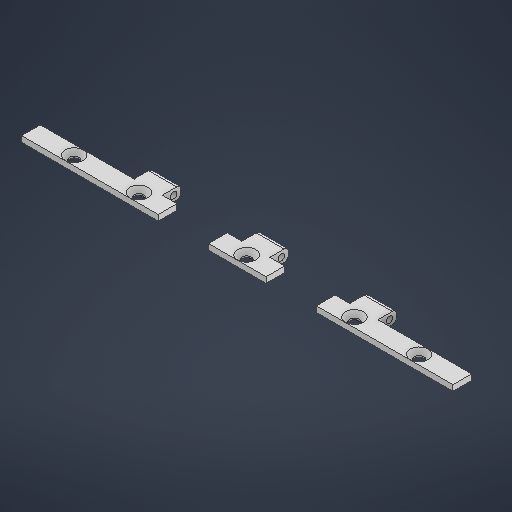
# Autodesk Inventor part: mocowanie do pługu
Saved by Autodesk Inventor 2026.2 (Build 302298010, 298A)
## iProperties
Created: 2026-05-09
Part Number: mocowanie do pługu
Material: Ogólny
Document SubType Name: Modeling
Designer: karol
Density: 1 g/cm^3
Appearance: Domyślna
Author: karol
Autodesk Inventor part; units mm, degrees
ref_plane "YZ Plane" through (0, 0, 0) normal (1, 0, 0) x (0, 1, 0)
ref_plane "XZ Plane" through (0, 0, 0) normal (0, 1, 0) x (-1, 0, 0)
ref_plane "XY Plane" through (0, 0, 0) normal (0, 0, 1) x (1, 0, 0)
sketch "Szkic1" plane through (0, 0, 0) normal (0, 1, 0) x (-1, 0, 0)
  line L0 (0, 0) -> (-4.9, 0)
  line L1 (-4.9, 0) -> (4.9, 0)
  line L2 (4.9, 0) -> (-4.8, 0)
  line L3 (-4.8, 0) -> (-4.8, -4.8)
  line L4 (-4.8, -4.8) -> (4.9, -4.8)
  line L5 (4.9, -4.8) -> (4.9, 0)
  line L6 (0, 0) -> (-37.5, 0)
  line L7 (0, 0) -> (37.5, 0)
  line L8 (37.5, 0) -> (32.6, 0)
  line L9 (37.5, 0) -> (42.4, 0)
  line L10 (-37.5, 0) -> (-32.6, 0)
  line L11 (-32.6, 0) -> (-42.4, 0)
  line L12 (42.4, 0) -> (32.6, 0)
  line L13 (32.6, 0) -> (32.6, -4.8)
  line L14 (32.6, -4.8) -> (42.4, -4.8)
  line L15 (42.4, -4.8) -> (42.4, 0)
  line L16 (-32.6, 0) -> (-42.4, 0)
  line L17 (-42.4, 0) -> (-42.4, -4.8)
  line L18 (-42.4, -4.8) -> (-32.6, -4.8)
  line L19 (-32.6, -4.8) -> (-32.6, 0)
  point P0 (-4.8, 0)
  dimension "d0" = 4.9
  dimension "d1" = 9.8
  dimension "d2" = 4.8
  dimension "d3" = 37.5
  dimension "d4" = 37.5
  dimension "d5" = 4.9
  dimension "d6" = 4.9
  dimension "d7" = 4.9
  dimension "d8" = 9.8
  constraints: 40 end point, 7 point on line, 6 parallel, 5 horizontal, 3 perpendicular
  measures "d0" distance of L0.start L0.end
  measures "d1" distance of L0.end L1.end
  measures "d2" distance of L3.end L2.end
  measures "d3" distance of L0.start L6.end
  measures "d4" distance of L0.start L7.end
  measures "d5" distance of L7.end L8.end
  measures "d6" distance of L7.end L9.end
  measures "d7" distance of L6.end L10.end
  measures "d8" distance of L10.end L11.end
extrude "Wyciągnięcie proste1" add sketch "Szkic1" along normal blind 4
sketch "Szkic2" plane through (-32.6, 0, 0) normal (1, 0, 0) x (0, 0, -1)
  circle A0 centre (2.4, 2) radius 1.15
  line L0 (0, 4) -> (4.8, 4) projected
  line L1 (4.8, 0) -> (4.8, 4) projected
  point P0 (0, 0)
  dimension "d11" = 2.3
  dimension "d12" = 2
  dimension "d13" = 2.4
  constraints: 1 centre point
  measures "d11" diameter of A0
  measures "d12" distance from line of L0 A0.centre
  measures "d13" distance from line of L1 A0.centre
sketch "Szkic3" plane through (4.8, 0, 0) normal (1, 0, 0) x (0, 0, -1)
  circle A0 centre (2.4, 2) radius 1.15
  line L0 (4.8, 0) -> (4.8, 4) projected
  line L1 (0, 4) -> (4.8, 4) projected
  point P0 (0, 0)
  dimension "d14" = 2.3
  dimension "d15" = 2.4
  dimension "d16" = 2
  constraints: 1 centre point
  measures "d14" diameter of A0
  measures "d15" distance from line of L0 A0.centre
  measures "d16" distance from line of L1 A0.centre
sketch "Szkic4" plane through (42.4, 0, 0) normal (1, 0, 0) x (0, 0, -1)
  circle A0 centre (2.4, 2) radius 1.15
  line L0 (0, 4) -> (4.8, 4) projected
  line L1 (4.8, 0) -> (4.8, 4) projected
  point P0 (0, 0)
  dimension "d17" = 2.3
  dimension "d18" = 2
  dimension "d19" = 2.4
  constraints: 1 centre point
  measures "d17" diameter of A0
  measures "d18" distance from line of L0 A0.centre
  measures "d19" distance from line of L1 A0.centre
extrude "Wyciągnięcie proste2" cut sketch "Szkic4" against normal blind 9.8
extrude "Wyciągnięcie proste3" cut sketch "Szkic3" against normal blind 9.8
extrude "Wyciągnięcie proste4" cut sketch "Szkic2" against normal blind 9.8
fillet "Zaokrąglenie1" radius 1.25 6 edges at (-0.05, 4, -4.8) (-37.5, 4, -4.8) (37.5, 4, -4.8) (-0.05, 0, -4.8) (37.5, 0, -4.8) (-37.5, 0, -4.8)
sketch "Szkic11" plane through (-42.4, 4, 0) normal (0, 0, 1) x (1, 0, 0)
  line L0 (0, 0) -> (9.8, 0) projected
  line L1 (0, 0) -> (9.8, 0)
  line L2 (9.8, 0) -> (9.8, -4)
  line L3 (9.8, -4) -> (0, -4)
  line L4 (0, -4) -> (0, 0)
  line L5 (37.5, 0) -> (47.2, 0) projected
  line L6 (47.2, -4) -> (47.2, 0) projected
  line L7 (37.5, 0) -> (47.2, 0)
  line L8 (47.2, 0) -> (47.2, -4)
  line L9 (47.2, -4) -> (37.5, -4)
  line L10 (37.5, -4) -> (37.5, 0)
  line L11 (75, 0) -> (84.8, 0) projected
  line L12 (84.8, -4) -> (84.8, 0) projected
  line L13 (75, 0) -> (84.8, 0)
  line L14 (84.8, 0) -> (84.8, -4)
  line L15 (84.8, -4) -> (75, -4)
  line L16 (75, -4) -> (75, 0)
  point P0 (42.4, -4)
  point P1 (47.2, -2)
  point P2 (84.8, -2)
  point P3 (84.8, -2)
  point P4 (47.2, -2)
  constraints: 24 end point, 6 parallel, 3 horizontal, 3 perpendicular
extrude "Wyciągnięcie proste11" add sketch "Szkic11" against normal blind 6.5
sketch "Szkic12" plane through (-42.4, 0, 0) normal (-1, 0, 0) x (0, 0, 1)
  line L0 (0, 4) -> (-6.5, 4) projected
  line L1 (0, 0) -> (-6.5, 0) projected
  line L2 (-6.5, 4) -> (-1.5, 4)
  line L3 (-1.5, 4) -> (-1.5, 0)
  line L4 (-1.5, 0) -> (-6.5, 0)
  line L5 (-6.5, 0) -> (-6.5, 4)
  circle A0 centre (-4, 2) radius 1.1
  point P0 (-6.5, 2)
  dimension "d73" = 5
  dimension "d74" = 2.2
  dimension "d75" = 2
  dimension "d76" = 2.5
  constraints: 8 end point, 2 parallel, 1 centre point, 1 horizontal, 1 midpoint, 1 perpendicular, 1 point on line
  measures "d73" distance of L3.end L4.end
  measures "d74" diameter of A0
  measures "d75" distance from line of L0 A0.centre
  measures "d76" distance of point (-6.5, 2) A0.centre
sketch "Szkic13" plane through (-4.9, 0, 0) normal (-1, 0, 0) x (0, 0, 1)
  line L0 (0, 4) -> (-6.5, 4) projected
  line L1 (0, 0) -> (-6.5, 0) projected
  line L2 (-6.5, 4) -> (-1.5, 4)
  line L3 (-1.5, 4) -> (-1.5, 0)
  line L4 (-1.5, 0) -> (-6.5, 0)
  line L5 (-6.5, 0) -> (-6.5, 4)
  circle A0 centre (-4, 2) radius 1.1
  dimension "d77" = 5
  dimension "d78" = 2.2
  dimension "d79" = 2
  dimension "d80" = 2.5
  constraints: 8 end point, 2 parallel, 1 centre point, 1 horizontal, 1 perpendicular, 1 point on line
  measures "d77" distance of L3.end L4.end
  measures "d78" diameter of A0
  measures "d79" distance from line of L0 A0.centre
  measures "d80" distance from line of L5 A0.centre
sketch "Szkic14" plane through (32.6, 0, 0) normal (-1, 0, 0) x (0, 0, 1)
  line L0 (0, 4) -> (-6.5, 4) projected
  line L1 (0, 0) -> (-6.5, 0) projected
  line L2 (-6.5, 4) -> (-1.5, 4)
  line L3 (-1.5, 4) -> (-1.5, 0)
  line L4 (-1.5, 0) -> (-6.5, 0)
  line L5 (-6.5, 0) -> (-6.5, 4)
  circle A0 centre (-4, 2) radius 1.1
  dimension "d81" = 5
  dimension "d82" = 2.2
  dimension "d83" = 2
  dimension "d84" = 2.5
  constraints: 8 end point, 2 parallel, 1 centre point, 1 horizontal, 1 perpendicular, 1 point on line
  measures "d81" distance of L3.end L4.end
  measures "d82" diameter of A0
  measures "d83" distance from line of L0 A0.centre
  measures "d84" distance from line of L5 A0.centre
extrude "Wyciągnięcie proste12" cut sketch "Szkic14" against normal blind 10 contours A0
extrude "Wyciągnięcie proste13" cut sketch "Szkic13" against normal blind 10 contours A0
extrude "Wyciągnięcie proste14" cut sketch "Szkic12" against normal blind 10 contours A0
fillet "Zaokrąglenie4" radius 1.5 6 edges at (-37.5, 4, -6.5) (-0.05, 0, -6.5) (-0.05, 4, -6.5) (-37.5, 0, -6.5) (37.5, 0, -6.5) (37.5, 4, -6.5)
sketch "Szkic15" plane through (-42.4, 0, 0) normal (0, 0, 1) x (1, 0, 0)
  line L0 (0, 4) -> (9.8, 4) projected
  line L1 (9.8, 0) -> (9.8, 4) projected
  line L2 (0, 4) -> (9.8, 4)
  line L3 (9.8, 4) -> (9.8, 2)
  line L4 (9.8, 2) -> (0, 2)
  line L5 (0, 2) -> (0, 4)
  line L6 (9.8, 4) -> (4.9, 4)
  line L7 (4.9, 4) -> (4.9, 2)
  line L8 (4.9, 2) -> (9.8, 2)
  line L9 (9.8, 2) -> (9.8, 4)
  line L10 (4.9, 4) -> (14.9, 4)
  line L11 (14.9, 4) -> (14.9, 2)
  line L12 (14.9, 2) -> (4.9, 2)
  line L13 (4.9, 2) -> (4.9, 4)
  line L14 (4.9, 4) -> (-5.1, 4)
  line L15 (-5.1, 4) -> (-5.1, 2)
  line L16 (-5.1, 2) -> (4.9, 2)
  line L17 (4.9, 2) -> (4.9, 4)
  line L18 (37.5, 0) -> (37.5, 4) projected
  line L19 (47.2, 0) -> (47.2, 4) projected
  line L20 (37.5, 4) -> (47.2, 4)
  line L21 (47.2, 4) -> (47.2, 2)
  line L22 (47.2, 2) -> (37.5, 2)
  line L23 (37.5, 2) -> (37.5, 4)
  line L24 (37.5, 4) -> (42.4, 4)
  line L25 (42.4, 4) -> (42.4, 2)
  line L26 (42.4, 2) -> (37.5, 2)
  line L27 (37.5, 2) -> (37.5, 4)
  line L28 (42.4, 4) -> (52.4, 4)
  line L29 (52.4, 4) -> (52.4, 2)
  line L30 (52.4, 2) -> (42.4, 2)
  line L31 (42.4, 2) -> (42.4, 4)
  line L32 (42.4, 4) -> (32.4, 4)
  line L33 (32.4, 4) -> (32.4, 2)
  line L34 (32.4, 2) -> (42.4, 2)
  line L35 (42.4, 2) -> (42.4, 4)
  line L36 (84.8, 0) -> (84.8, 4) projected
  line L37 (75, 0) -> (75, 4) projected
  line L38 (84.8, 4) -> (75, 4)
  line L39 (75, 4) -> (75, 2)
  line L40 (75, 2) -> (84.8, 2)
  line L41 (84.8, 2) -> (84.8, 4)
  line L42 (75, 4) -> (79.9, 4)
  line L43 (79.9, 4) -> (79.9, 2)
  line L44 (79.9, 2) -> (75, 2)
  line L45 (75, 2) -> (75, 4)
  line L46 (79.9, 4) -> (69.9, 4)
  line L47 (69.9, 4) -> (69.9, 2)
  line L48 (69.9, 2) -> (79.9, 2)
  line L49 (79.9, 2) -> (79.9, 4)
  line L50 (79.9, 4) -> (89.9, 4)
  line L51 (89.9, 4) -> (89.9, 2)
  line L52 (89.9, 2) -> (79.9, 2)
  line L53 (79.9, 2) -> (79.9, 4)
  line L54 (89.9, 4) -> (122.4, 4)
  line L55 (122.4, 4) -> (122.4, 2)
  line L56 (122.4, 2) -> (89.9, 2)
  line L57 (89.9, 2) -> (89.9, 4)
  line L58 (-5.1, 4) -> (-37.6, 4)
  line L59 (-37.6, 4) -> (-37.6, 2)
  line L60 (-37.6, 2) -> (-5.1, 2)
  line L61 (-5.1, 2) -> (-5.1, 4)
  point P0 (42.4, 0)
  dimension "d92" = 10
  dimension "d93" = 10
  dimension "d94" = 10
  dimension "d95" = 10
  dimension "d96" = 10
  dimension "d97" = 10
  dimension "d98" = 32.5
  dimension "d99" = 32.5
  constraints: 112 end point, 28 parallel, 14 horizontal, 14 perpendicular, 7 point on line, 5 midpoint
  measures "d92" distance of L11.end L12.end
  measures "d93" distance of L16.end L15.end
  measures "d94" distance of L29.end L30.end
  measures "d95" distance of L34.end L33.end
  measures "d96" distance of L48.end L47.end
  measures "d97" distance of L51.end L52.end
  measures "d98" distance of L55.end L56.end
  measures "d99" distance of L60.end L59.end
extrude "Wyciągnięcie proste15" add sketch "Szkic15" along normal blind 6.5
sketch "Szkic17" plane through (-80, 2, 0) normal (-1, 0, 0) x (0, 0, 1)
  line L0 (0, 0) -> (6.5, 0) projected
  line L1 (0, 0) -> (6.5, 0)
  line L2 (6.5, 0) -> (6.5, 2)
  line L3 (6.5, 2) -> (0, 2)
  line L4 (0, 2) -> (0, 0)
  point P0 (0, -2)
  point P1 (6.5, 0)
  constraints: 8 end point, 2 parallel, 1 horizontal, 1 perpendicular
extrude "Wyciągnięcie proste16" cut sketch "Szkic17" against normal blind 5
sketch "Szkic18" plane through (80, 2, 0) normal (1, 0, 0) x (0, 0, -1)
  line L0 (0, 0) -> (-6.5, 0) projected
  line L1 (-6.5, 0) -> (-6.5, 2) projected
  line L2 (0, 0) -> (-6.5, 0)
  line L3 (-6.5, 0) -> (-6.5, 2)
  line L4 (-6.5, 2) -> (0, 2)
  line L5 (0, 2) -> (0, 0)
  point P0 (0, -2)
  constraints: 8 end point, 2 parallel, 1 horizontal, 1 perpendicular
extrude "Wyciągnięcie proste17" cut sketch "Szkic18" against normal blind 5
sketch "Szkic19" plane through (0, 4, 0) normal (0, 1, 0) x (1, 0, 0)
  circle A0 centre (0, -3.25) radius 1.5265
  line L0 (10, -6.5) -> (-10, -6.5) projected
  line L1 (10, 0) -> (10, -6.5) projected
  circle A1 centre (-60, -3.25) radius 0.8171
  circle A2 centre (-37.5, -3.25) radius 1.1163
  circle A3 centre (60, -3.25) radius 1.1244
  circle A4 centre (37.5, -3.25) radius 1.6836
  line L2 (75, -6.5) -> (27.5, -6.5) projected
  line L3 (75, -6.5) -> (75, 0) projected
  line L4 (-75, 0) -> (-75, -6.5) projected
  line L5 (-27.5, -6.5) -> (-75, -6.5) projected
  point P0 (0, 0)
  point P1 (0, -6.5)
  point P2 (75, -3.25)
  point P3 (-75, -3.25)
  dimension "d123" = 3.25
  dimension "d124" = 10
  dimension "d125" = 3.25
  dimension "d126" = 3.25
  dimension "d127" = 15
  dimension "d128" = 37.5
  dimension "d129" = 37.5
  dimension "d130" = 15
  dimension "d131" = 3.25
  dimension "d132" = 3.25
  constraints: 5 centre point, 3 midpoint
  measures "d123" distance of point (0, -6.5) A0.centre
  measures "d124" distance from line of L1 A0.centre
  measures "d125" distance from line of L2 A4.centre
  measures "d126" distance from line of L2 A3.centre
  measures "d127" distance of A3.centre point (75, -3.25)
  measures "d128" distance from line of L3 A4.centre
  measures "d129" distance of A2.centre point (-75, -3.25)
  measures "d130" distance from line of L4 A1.centre
  measures "d131" distance from line of L5 A1.centre
  measures "d132" distance from line of L5 A2.centre
hole "Otwór3" at (-60, 4, 3.25) at (-37.5, 4, 3.25) at (0, 4, 3.25) at (37.5, 4, 3.25) at (60, 4, 3.25) direction (0, -1, 0) diameter 3.3 depth 2 tip angle 118 countersink diameter 6.3 countersink angle 90
